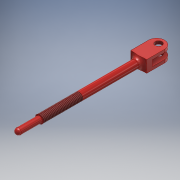
# Autodesk Inventor part: reverse gear steam chest rod valve 1
Saved by Autodesk Inventor 2017 (Build 210142000, 142)
## iProperties
Created: 2018-11-05
Part Number: reverse gear steam chest rod valve 1
Material: Generic
Document SubType Name: Modeling
Designer: User
Density: 1 g/cm^3
Appearance: Default
Author: User
Autodesk Inventor part; units mm, degrees
ref_plane "YZ Plane" through (0, 0, 0) normal (1, 0, 0) x (0, 1, 0)
ref_plane "XZ Plane" through (0, 0, 0) normal (0, 1, 0) x (-1, 0, 0)
ref_plane "XY Plane" through (0, 0, 0) normal (0, 0, 1) x (1, 0, 0)
sketch "Sketch1" plane through (0, 0, 0) normal (0, 1, 0) x (-1, 0, 0)
  circle A0 centre (0, 0) radius 1.5
  dimension "d0" = 3
  constraints: 1 centre point, 1 coincident
  measures "d0" diameter of A0
extrude "Extrusion1" add sketch "Sketch1" along normal blind 12
sketch "Sketch2" plane through (0, 12, 0) normal (0, 1, 0) x (1, 0, 0)
  circle A0 centre (0, 0) radius 2
  dimension "d3" = 4
  constraints: 1 centre point, 1 coincident
  measures "d3" diameter of A0
extrude "Extrusion2" add sketch "Sketch2" along normal blind 50
thread "Thread1" size "M4x0.7" class "6g" standard "ANSI Metric M Profile" length 20.5 offset 30
fillet "Fillet1" radius 1.5 1 edges at (1.5, 0, 0)
sketch "Sketch6" plane through (0, 62, 0) normal (0, 1, 0) x (1, 0, 0)
  line L0 (4, 3) -> (-4, 3)
  line L1 (-4, 3) -> (-4, -3)
  line L2 (-4, -3) -> (4, -3)
  line L3 (4, -3) -> (4, 3)
  line L4 (4, 3) -> (-4, -3) construction
  line L5 (-4, 3) -> (4, -3) construction
  point P0 (0, 0)
  point P1 (0, 0)
  dimension "d49" = 8
  dimension "d50" = 6
  dimension "d51" = 4
  dimension "d52" = 3
  dimension "d53" = 4
  dimension "d54" = 3
  constraints: 12 end point, 2 parallel, 1 horizontal, 1 perpendicular
  measures "d49" distance of L2.end L1.end
  measures "d50" distance of L1.end L0.end
  measures "d51" distance from line of point (0, 0) L3
  measures "d52" distance from line of point (0, 0) L0
  measures "d53" distance from line of point (0, 0) L3
  measures "d54" distance from line of point (0, 0) L0
extrude "Extrusion6" add sketch "Sketch6" along normal blind 3
sketch "Sketch7" plane through (0, 65, 0) normal (0, 1, 0) x (1, 0, 0)
  line L0 (-4, -3) -> (4, -3)
  line L1 (4, -3) -> (4, -1.5)
  line L2 (4, -1.5) -> (-4, -1.5)
  line L3 (-4, -1.5) -> (-4, -3)
  line L4 (4, 3) -> (-4, 3)
  line L5 (-4, 3) -> (4, 3)
  line L6 (4, 3) -> (4, 1.5)
  line L7 (4, 1.5) -> (-4, 1.5)
  line L8 (-4, 1.5) -> (-4, 3)
  point P0 (0, 0)
  point P1 (0, 0)
  dimension "d57" = 1.5
  dimension "d58" = 1.5
  dimension "d59" = 4.5
  dimension "d60" = 8
  dimension "d61" = 8
  dimension "d62" = 3
  dimension "d63" = 4
  dimension "d64" = 0
  dimension "d65" = 4
  dimension "d66" = 3
  constraints: 18 end point, 5 parallel, 2 horizontal, 2 perpendicular, 1 point on line
  measures "d57" distance of L1.end L0.end
  measures "d58" distance of L5.end L6.end
  measures "d59" distance between parallel lines of L5 L2
  measures "d60" distance between parallel lines of L8 L1
  measures "d61" distance between parallel lines of L1 L3
  measures "d62" distance from line of point (0, 0) L5
  measures "d63" distance from line of point (0, 0) L1
  measures "d64" distance from line of L4.start L1
  measures "d65" distance from line of point (0, 0) L1
  measures "d66" distance from line of point (0, 0) L5
extrude "Extrusion7" add sketch "Sketch7" along normal blind 10
sketch "Sketch8" plane through (4, 62, -3) normal (0, 0, -1) x (-1, 0, 0)
  line L0 (8, 0) -> (0, 0)
  circle A0 centre (4, 10) radius 1.75
  point P0 (4, -62)
  point P1 (4, -62)
  dimension "d69" = 3.5
  dimension "d70" = 62
  dimension "d71" = 10
  dimension "d72" = 62
  dimension "d73" = 62.1289
  dimension "d74" = 72
  dimension "d75" = 0
  dimension "d76" = 62.1289
  constraints: 2 end point, 1 centre point, 1 horizontal
  measures "d69" diameter of A0
  measures "d70" distance from line of point (4, -62) L0
  measures "d71" distance from line of A0.centre L0
  measures "d72" distance from line of point (4, -62) L0
  measures "d73" distance of point (4, -62) L0.start
  measures "d74" distance of point (4, -62) A0.centre
  measures "d75" distance of point (4, -62) point (4, -62)
  measures "d76" distance of point (4, -62) L0.end
extrude "Extrusion8" cut sketch "Sketch8" against normal through all
fillet "Fillet5" radius 4 4 edges at (-4, 75, -2.25) (-4, 75, 2.25) (4, 75, -2.25) (4, 75, 2.25)
fillet "Fillet6" radius 2 1 edges at (-2, 62, 0)
body "Solid1"
